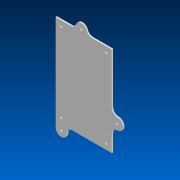
# Autodesk Inventor part: PDP Mount
Saved by Autodesk Inventor 2022 (Build 260153000, 153)
## iProperties
Created: 2022-04-13
Part Number: PDP Mount
Material: Generic
Document SubType Name: Modeling
Designer: score_nygvs6w
Density: 1 g/cm^3
Appearance: Default
Author: score_nygvs6w
Autodesk Inventor part; units mm, degrees
ref_plane "YZ Plane" through (0, 0, 0) normal (1, 0, 0) x (0, 1, 0)
ref_plane "XZ Plane" through (0, 0, 0) normal (0, 1, 0) x (-1, 0, 0)
ref_plane "XY Plane" through (0, 0, 0) normal (0, 0, 1) x (1, 0, 0)
sketch "Sketch1" plane through (0, 0, 0) normal (0, 0, 1) x (1, 0, 0)
  line L0 (50.8, 88.9) -> (-50.8, 88.9) construction
  line L1 (-50.8, 88.9) -> (-50.8, -88.9) construction
  line L2 (-50.8, -88.9) -> (50.8, -88.9) construction
  line L3 (50.8, -88.9) -> (50.8, 88.9) construction
  line L4 (50.8, 88.9) -> (-50.8, -88.9) construction
  line L5 (-50.8, 88.9) -> (50.8, -88.9) construction
  line L6 (-63.5, -101.6) -> (63.5, -101.6)
  line L7 (63.5, -101.6) -> (63.5, 101.6)
  line L8 (63.5, 101.6) -> (-63.5, 101.6)
  line L9 (-63.5, 101.6) -> (-63.5, -101.6)
  line L10 (-63.5, -101.6) -> (63.5, 101.6) construction
  line L11 (63.5, -101.6) -> (-63.5, 101.6) construction
  circle A0 centre (-4.9961, 106.596) radius 12.7
  circle A1 centre (76.2, -38.1) radius 12.7
  circle A2 centre (-50.8, -114.3) radius 12.7
  arc A3 (-29.1996, 101.6) -> (-17.0978, 110.448) centre (-29.1996, 114.3) ccw
  arc A4 (7.1056, 110.448) -> (19.2074, 101.6) centre (19.2074, 114.3) ccw
  arc A5 (63.5, -12.7) -> (76.2, -25.4) centre (76.2, -12.7) ccw
  arc A6 (76.2, -50.8) -> (63.5, -63.5) centre (76.2, -63.5) ccw
  arc A7 (-25.4, -101.6) -> (-38.1, -114.3) centre (-25.4, -114.3) ccw
  line L12 (-63.5, -114.3) -> (-63.5, -101.6)
  point P0 (0, 0)
  point P1 (-50.8, -101.6)
  dimension "d0" = 101.6
  dimension "d1" = 177.8
  dimension "d2" = 12.7
  dimension "d3" = 12.7
  dimension "d13" = 25.4
  dimension "d16" = 127
  dimension "d17" = 76.2
  constraints: 26 end point, 16 point on circle, 12 tangent, 8 centre point, 7 coincident, 7 equal radius, 5 point on line, 4 midpoint, 4 parallel, 2 horizontal, 2 perpendicular, 1 vertical
  measures "d0" distance of L2.end L1.end
  measures "d1" distance of L1.end L0.end
  measures "d2" distance between parallel lines of L0 L8
  measures "d3" distance between parallel lines of L9 L1
  measures "d13" diameter of A0
  measures "d16" horizontal distance of point (76.2, -38.1) point (-50.8, -114.3)
  measures "d17" vertical distance of point (-50.8, -114.3) point (76.2, -38.1)
extrude "Extrusion1" add sketch "Sketch1" along normal blind 3.175
hole "Hole1" at (-50.8, 88.9, 0) at (50.8, 88.9, 0) at (50.8, -88.9, 0) at (-50.8, -88.9, 0) at (-50.8, -114.3, 0) at (76.2, -38.1, 0) at (-4.9961, 106.596, 0) direction (0, 0, 1) diameter 4.572 end through all
body "Solid1"
